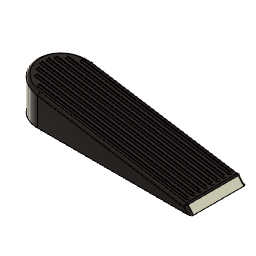
Door Stop (Autodesk Fusion 360 design; units mm, degrees)
Autodesk Fusion 360 part; units mm, degrees
box "BoxPrimitive1" add length 45.72 width 127 height 5.08 placed x (0, 1, 0) y (-1, 0, 0) z (0, 0, 1) at (127, 0, 0)
cylinder "CylinderPrimitive1" add diameter 45.72 height -5.08 placed x (1, 0, 0) y (0, 1, 0) z (0, 0, 1) at (0, 22.86, 5.08)
draft "Draft1" angle 9 neutral plane through (127, 0, 0) pull (1, 0, 0) 1 faces at (84.6667, 15.24, 5.08)
chamfer "Chamfer1" distance 5.08 angle 45 1 edges at (127, 22.86, 5.08)
shell "Shell1" thickness 2.54 removed faces 2 at (127, 30.48, 0.0003) at (84.6667, 15.24, 0)
fillet "Fillet1" radius 2.032 6 edges at (60.9913, 45.72, 15.5348) (-22.86, 22.86, 28.8155) (60.9913, 0, 15.5348) (121.9825, 22.86, 5.8747) (124.4913, 0, 2.9373) (124.4913, 45.72, 2.9373)
sketch "Sketch3" plane through (3.8928, 0, 24.5783) normal (0.156434, 0, 0.987688) x (0, 1, 0)
  line L0 (43.688, -118.8121) -> (43.688, 3.6195)
  ellipse E0 centre (22.86, 3.6195) end of major axis (22.86, 24.7071) minor radius 20.828 (43.688, 3.6195) -> (2.032, 3.6195) ccw
  line L1 (2.032, 3.6195) -> (2.032, -118.8121)
  line L2 (2.032, -118.8121) -> (43.688, -118.8121)
  line L3 (6.35, -116.078) -> (6.35, 30.48)
  line L4 (6.35, 30.48) -> (3.81, 30.48)
  line L5 (3.81, 30.48) -> (3.81, -116.078)
  arc A0 (3.81, -116.078) -> (6.35, -116.078) centre (5.08, -116.078) ccw
  line L6 (11.43, -116.078) -> (11.43, 30.48)
  line L7 (8.89, 30.48) -> (8.89, -116.078)
  arc A1 (8.89, -116.078) -> (11.43, -116.078) centre (10.16, -116.078) ccw
  line L8 (11.43, 30.48) -> (8.89, 30.48)
  line L9 (16.51, -116.078) -> (16.51, 30.48)
  line L10 (13.97, 30.48) -> (13.97, -116.078)
  arc A2 (13.97, -116.078) -> (16.51, -116.078) centre (15.24, -116.078) ccw
  line L11 (16.51, 30.48) -> (13.97, 30.48)
  line L12 (21.59, -116.078) -> (21.59, 30.48)
  line L13 (19.05, 30.48) -> (19.05, -116.078)
  arc A3 (19.05, -116.078) -> (21.59, -116.078) centre (20.32, -116.078) ccw
  line L14 (21.59, 30.48) -> (19.05, 30.48)
  circle A4 centre (5.08, 7.549) radius 1.27
  circle A5 centre (10.16, 15.0787) radius 1.27
  circle A6 centre (15.24, 18.8436) radius 1.27
  circle A7 centre (20.32, 20.8367) radius 1.27
  line L15 (22.86, -118.8121) -> (22.86, 24.7071) construction
  line L16 (24.13, 30.48) -> (26.67, 30.48)
  line L17 (34.29, 30.48) -> (36.83, 30.48)
  line L18 (31.75, 30.48) -> (31.75, -116.078)
  circle A8 centre (40.64, 7.549) radius 1.27
  circle A9 centre (30.48, 18.8436) radius 1.27
  arc A10 (39.37, -116.078) -> (41.91, -116.078) centre (40.64, -116.078) ccw
  line L19 (39.37, -116.078) -> (39.37, 30.48)
  line L20 (29.21, 30.48) -> (31.75, 30.48)
  arc A11 (34.29, -116.078) -> (36.83, -116.078) centre (35.56, -116.078) ccw
  line L21 (34.29, -116.078) -> (34.29, 30.48)
  line L22 (24.13, -116.078) -> (24.13, 30.48)
  line L23 (43.688, 3.6195) -> (43.688, -118.8121)
  line L24 (29.21, -116.078) -> (29.21, 30.48)
  arc A12 (29.21, -116.078) -> (31.75, -116.078) centre (30.48, -116.078) ccw
  line L25 (36.83, 30.48) -> (36.83, -116.078)
  arc A13 (24.13, -116.078) -> (26.67, -116.078) centre (25.4, -116.078) ccw
  circle A14 centre (35.56, 15.0787) radius 1.27
  circle A15 centre (25.4, 20.8367) radius 1.27
  line L26 (26.67, 30.48) -> (26.67, -116.078)
  line L27 (39.37, 30.48) -> (41.91, 30.48)
  line L28 (41.91, 30.48) -> (41.91, -116.078)
  point P0 (45.72, 0)
  dimension "d16" = 15.24
  dimension "d17" = 0
  constraint vertical L3
  constraint horizontal L4
  constraint vertical L5
  constraint tangent L5 A4
  constraint tangent L3 A4
  constraint tangent L7 A5
  constraint tangent L6 A5
  constraint tangent L10 A6
  constraint tangent L9 A6
  constraint tangent L13 A7
  constraint tangent L12 A7
  constraint midpoint L2 L15.start
  constraint coincident E0 L15.end
  constraint perpendicular L2 L15
  constraint symmetric origin L15 P0
  constraint symmetric L1.start L15 L0.end
  constraint symmetric L1.end L15 L0.start
  constraint symmetric L5.end L15 A10.end
  constraint symmetric L3.start L15 A10.start
  constraint symmetric L3.end L15 L19.end
  constraint symmetric L4.end L15 L27.end
  constraint symmetric A0 L15 A10
  constraint symmetric L6.start L15 A11.start
  constraint symmetric L6.end L15 L17.start
  constraint symmetric L7.start L15 L17.end
  constraint symmetric L7.end L15 A11.end
  constraint symmetric A1 L15 A11
  constraint symmetric L9.start L15 L24.start
  constraint symmetric L9.end L15 L20.start
  constraint symmetric L10.start L15 L18.start
  constraint symmetric L10.end L15 L18.end
  constraint symmetric A2 L15 A12
  constraint symmetric L12.start L15 L22.start
  constraint symmetric L12.end L15 L16.start
  constraint symmetric L13.start L15 L16.end
  constraint symmetric L13.end L15 A13.end
  constraint symmetric A3 L15 A13
  constraint symmetric A4 L15 A8
  constraint symmetric A5 L15 A14
  constraint symmetric A6 L15 A9
  constraint symmetric A7 L15 A15
extrude "Extrude1" add sketch "Sketch3" along normal blind 1.27 contours A8 | A8 A10 L19 L28 | L3 L5 A0 A4 | A4 | A14 | A11 L21 L25 A14 | L6 L7 A1 A5 | A5 | A9 | L18 A9 L24 A12 | L9 L10 A2 A6 | A6 | A15 | L22 A13 A15 L26 | L12 L13 A3 A7 | A7
fillet "Fillet2" radius 1.016 32 edges at (57.6879, 6.35, 17.3438) (-4.619, 5.08, 27.2122) (57.6879, 3.81, 17.3438) (119.9947, 5.08, 7.4754) (53.9694, 11.43, 17.9327) (-12.056, 10.16, 28.3901) (53.9694, 8.89, 17.9327) (119.9947, 10.16, 7.4754) (52.1101, 16.51, 18.2272) (-15.7744, 15.24, 28.9791) (52.1101, 13.97, 18.2272) (119.9947, 15.24, 7.4754) (51.1258, 21.59, 18.3831) (-17.7431, 20.32, 29.2909) (51.1258, 19.05, 18.3831) (119.9947, 20.32, 7.4754) (51.1258, 26.67, 18.3831) (-17.7431, 25.4, 29.2909) (51.1258, 24.13, 18.3831) (119.9947, 25.4, 7.4754) (52.1101, 29.21, 18.2272) (119.9947, 30.48, 7.4754) (52.1101, 31.75, 18.2272) (-15.7744, 30.48, 28.9791) (53.9694, 34.29, 17.9327) (119.9947, 35.56, 7.4754) (53.9694, 36.83, 17.9327) (-12.056, 35.56, 28.3901) (57.6879, 41.91, 17.3438) (-4.619, 40.64, 27.2122) (57.6879, 39.37, 17.3438) (119.9947, 40.64, 7.4754)
